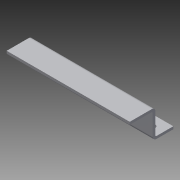
# Autodesk Inventor part: Chassis Battery Mount Part1
Saved by Autodesk Inventor 2013 (Build 170138000, 138)
## iProperties
Created: 2013-01-24
Part Number: Chassis Battery Mount Part1
Material: Aluminum 6061
Document SubType Name: Sheet Metal
Designer: Moses
Density: 2.71 g/cm^3
Sheet Metal Rule: Default
Mass: 107.425 g
Surface Area: 268.62 cm^2
Volume: 39.6403 cm^3
Author: Moses
Autodesk Inventor part; units mm, degrees
ref_plane "YZ Plane" through (0, 0, 0) normal (1, 0, 0) x (0, 1, 0)
ref_plane "XZ Plane" through (0, 0, 0) normal (0, 1, 0) x (-1, 0, 0)
ref_plane "XY Plane" through (0, 0, 0) normal (0, 0, 1) x (1, 0, 0)
sketch "Sketch1" plane through (0, 0, 0) normal (0, 1, 0) x (-1, 0, 0)
  line L0 (0, 0) -> (152.4, 0)
  line L1 (152.4, 0) -> (152.4, 25.4)
  line L2 (152.4, 25.4) -> (0, 25.4)
  line L3 (0, 25.4) -> (0, 0)
  line L4 (0, 12.7) -> (152.4, 12.7) construction
  circle A0 centre (12.7, 12.7) radius 3.302
  circle A1 centre (38.1, 12.7) radius 3.302
  circle A2 centre (63.5, 12.7) radius 3.302
  circle A3 centre (88.9, 12.7) radius 3.302
  circle A4 centre (114.3, 12.7) radius 3.302
  circle A5 centre (139.7, 12.7) radius 3.302
  dimension "d0" = 25.4
  dimension "d1" = 152.4
  dimension "d2" = 6.604
  dimension "d3" = 12.7
  dimension "d6" = 25.4
  dimension "d11" = 12.7
  measures "d0" distance of L2.end L0.start
  measures "d1" distance of L0.start L0.end
  measures "d2" diameter of A0
  measures "d3" distance from line of A0.centre L3
  measures "d6" distance of A0.centre A1.centre
  measures "d11" distance from line of L1 A5.centre
extrude "Plate1" add sketch "Sketch1" along normal blind 3.175
sketch "Sketch2" plane through (0, 0, 22.225) normal (0, 0, 1) x (1, 0, 0)
  line L0 (-152.4, 0) -> (0, 0)
  line L1 (0, 0) -> (0, 31.75)
  line L2 (0, 31.75) -> (-152.4, 31.75)
  line L3 (-152.4, 31.75) -> (-152.4, 0)
  constraints: 6 end point, 1 horizontal, 1 perpendicular, 1 vertical
edge flange "Flange1" height 31.75 angle 90 thickness 3.175 bend radius 1.27 thickness toward (0, 0, 1) relief straight relief width 3.175 relief depth 1.5875 edges at (-76.2, 3.175, 25.4) wall of the first edge with corners at (-152.4, 0, 22.225) (0, 0, 22.225) (0, 31.75, 22.225) (-152.4, 31.75, 22.225)
bend "Bend1"
corner "Corner1"
sketch "Sketch3" plane through (-152.4, 31.75, 25.4) normal (0, 1, 0) x (-1, 0, 0)
  line L0 (-152.4, 0) -> (0, 0)
  line L1 (0, 0) -> (0, 28.575)
  line L2 (0, 28.575) -> (-152.4, 28.575)
  line L3 (-152.4, 28.575) -> (-152.4, 0)
  constraints: 6 end point, 1 horizontal, 1 perpendicular, 1 vertical
edge flange "Flange2" height 31.75 angle 90 thickness 3.175 bend radius 1.27 thickness toward (0, 1, 0) relief straight relief width 3.175 relief depth 1.5875 edges at (-76.2, 31.75, 25.4) wall of the first edge with corners at (0, 31.75, 25.4) (-152.4, 31.75, 25.4) (-152.4, 31.75, 53.975) (0, 31.75, 53.975)
bend "Bend2"
corner "Corner2"
equation "\"d13\" = BendReliefWidth"
equation "\"d14\" = BendReliefDepth"
equation "\"d15\" = MinimumRemnant"
equation "\"d16\" = BendRadius"
equation "\"d20\" = CornerReliefSize"
equation "\"d21\" = GapSize"
equation "\"d22\" = JacobiRadiusSize"
equation "\"d23\" = BendReliefWidth"
equation "\"d24\" = BendReliefDepth"
equation "\"d25\" = MinimumRemnant"
equation "\"d26\" = BendRadius"
equation "\"d30\" = CornerReliefSize"
equation "\"d31\" = GapSize"
equation "\"d32\" = JacobiRadiusSize"
equation "\"BendRadius\" = Thickness"
equation "\"BendReliefWidth\" = Thickness"
equation "\"BendReliefDepth\" = 0.5 * Thickness"
equation "\"CornerReliefSize\" = 4 * Thickness"
equation "\"MinimumRemnant\" = 2 * Thickness"
equation "\"TransitionRadius\" = BendRadius"
equation "\"JacobiRadiusSize\" = BendRadius"
equation "\"GapSize\" = Thickness"
equation "\"d12\" = BendRadius"
equation "\"Thickness\" = 3.175"
body "Solid1"
